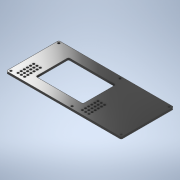
# Autodesk Inventor part: Sole_frame
Saved by Autodesk Inventor 2020.4 (Build 244396000, 396)
## iProperties
Part Number: Sole_frame
Material: GFRP
Document SubType Name: Modeling
Designer: Masato Kubotera
Density: 1.75 g/cm^3
Appearance: 低 光沢 - 黒
Description: GFRP T3
Mass: 61.6656 g
Surface Area: 261.936 cm^2
Volume: 35.2375 cm^3
Author: Masato Kubotera
Autodesk Inventor part; units mm, degrees
ref_plane "YZ Plane" through (0, 0, 0) normal (1, 0, 0) x (0, 1, 0)
ref_plane "XZ Plane" through (0, 0, 0) normal (0, 1, 0) x (-1, 0, 0)
ref_plane "XY Plane" through (0, 0, 0) normal (0, 0, 1) x (1, 0, 0)
sketch "スケッチ1" plane through (0, 0, 0) normal (0, 0, 1) x (1, 0, 0)
  line L0 (-96.735, 54.75) -> (78.265, 54.75)
  line L1 (78.265, 54.75) -> (78.265, -25.25)
  line L2 (78.265, -25.25) -> (-96.735, -25.25)
  line L3 (-96.735, -25.25) -> (-96.735, 54.75)
  line L4 (-96.735, 54.75) -> (78.265, -25.25) construction
  line L5 (78.265, 54.75) -> (-96.735, -25.25) construction
  line L6 (-96.735, 14.75) -> (78.265, 14.75) construction
  line L7 (-96.735, 0) -> (78.265, 0) construction
  line L8 (-80, 4.75) -> (-80, -4.75) construction
  circle A0 centre (-80, -4.75) radius 1.6
  line L9 (0, 54.75) -> (0, -25.25) construction
  line L10 (18, -4.75) -> (18, 4.75) construction
  circle A1 centre (18, -4.75) radius 1.6
  circle A2 centre (-80, 4.75) radius 1.6
  circle A3 centre (18, 4.75) radius 1.6
  line L11 (74.765, -21.75) -> (-93.235, -21.75) construction
  line L12 (-93.235, -21.75) -> (-93.235, 51.25) construction
  line L13 (-93.235, 51.25) -> (74.765, 51.25) construction
  line L14 (74.765, 51.25) -> (74.765, -21.75) construction
  line L15 (74.765, -21.75) -> (-93.235, 51.25) construction
  line L16 (-93.235, -21.75) -> (74.765, 51.25) construction
  circle A4 centre (-93.235, 51.25) radius 1.6
  circle A5 centre (0, 51.25) radius 1.6
  circle A6 centre (74.765, 51.25) radius 1.6
  circle A7 centre (-93.235, -21.75) radius 1.6
  circle A8 centre (0, -21.75) radius 1.6
  circle A9 centre (74.765, -21.75) radius 1.6
  line L17 (15, 12.5) -> (21, 12.5) construction
  line L18 (21, 12.5) -> (21, -12.5) construction
  line L19 (21, -12.5) -> (15, -12.5) construction
  line L20 (15, -12.5) -> (15, 12.5) construction
  line L21 (15, 12.5) -> (21, -12.5) construction
  line L22 (21, 12.5) -> (15, -12.5) construction
  line L23 (-83, 12.5) -> (-77, 12.5) construction
  line L24 (-77, 12.5) -> (-77, -12.5) construction
  line L25 (-77, -12.5) -> (-83, -12.5) construction
  line L26 (-83, -12.5) -> (-83, 12.5) construction
  line L27 (-83, 12.5) -> (-77, -12.5) construction
  line L28 (-77, 12.5) -> (-83, -12.5) construction
  line L29 (-67, 39.75) -> (5, 39.75)
  line L30 (5, 39.75) -> (5, -10.25)
  line L31 (5, -10.25) -> (-67, -10.25)
  line L32 (-67, -10.25) -> (-67, 39.75)
  line L33 (-67, 39.75) -> (5, -10.25) construction
  line L34 (5, 39.75) -> (-67, -10.25) construction
  circle A10 centre (-80, 0) radius 1.6
  circle A11 centre (18, 0) radius 1.6
  circle A12 centre (-80, -9.5) radius 1.6
  circle A13 centre (18, -9.5) radius 1.6
  circle A14 centre (-80, -4.75) radius 1.6
  circle A15 centre (18, -4.75) radius 1.6
  circle A16 centre (-80, -14.25) radius 1.6
  circle A17 centre (18, -14.25) radius 1.6
  circle A18 centre (-80, -9.5) radius 1.6
  circle A19 centre (18, -9.5) radius 1.6
  circle A20 centre (-80, -19) radius 1.6
  circle A21 centre (18, -19) radius 1.6
  circle A22 centre (-80, -14.25) radius 1.6
  circle A23 centre (18, -14.25) radius 1.6
  circle A24 centre (-85, 4.75) radius 1.6
  circle A25 centre (-85, 0) radius 1.6
  circle A26 centre (-85, -4.75) radius 1.6
  circle A27 centre (-85, -9.5) radius 1.6
  circle A28 centre (-85, -14.25) radius 1.6
  circle A29 centre (-85, -19) radius 1.6
  circle A30 centre (13, 4.75) radius 1.6
  circle A31 centre (13, 0) radius 1.6
  circle A32 centre (13, -4.75) radius 1.6
  circle A33 centre (13, -9.5) radius 1.6
  circle A34 centre (13, -14.25) radius 1.6
  circle A35 centre (13, -19) radius 1.6
  circle A36 centre (-75, 4.75) radius 1.6
  circle A37 centre (-75, 0) radius 1.6
  circle A38 centre (-75, -4.75) radius 1.6
  circle A39 centre (-75, -9.5) radius 1.6
  circle A40 centre (-75, -14.25) radius 1.6
  circle A41 centre (-75, -19) radius 1.6
  circle A42 centre (23, 4.75) radius 1.6
  circle A43 centre (23, 0) radius 1.6
  circle A44 centre (23, -4.75) radius 1.6
  circle A45 centre (23, -9.5) radius 1.6
  circle A46 centre (23, -14.25) radius 1.6
  circle A47 centre (23, -19) radius 1.6
  circle A48 centre (-80, 4.75) radius 1.6
  circle A49 centre (-80, 0) radius 1.6
  circle A50 centre (-80, -4.75) radius 1.6
  circle A51 centre (-80, -9.5) radius 1.6
  circle A52 centre (-80, -14.25) radius 1.6
  circle A53 centre (-80, -19) radius 1.6
  circle A54 centre (18, 4.75) radius 1.6
  circle A55 centre (18, 0) radius 1.6
  circle A56 centre (18, -4.75) radius 1.6
  circle A57 centre (18, -9.5) radius 1.6
  circle A58 centre (18, -14.25) radius 1.6
  circle A59 centre (18, -19) radius 1.6
  point P0 (0, 0)
  point P1 (-9.235, 14.75)
  point P2 (-80, 0)
  point P3 (18, 0)
  point P4 (-31, 14.75)
  dimension "d0" = 175
  dimension "d1" = 80
  dimension "d2" = 25.25
  dimension "d3" = 3.2
  dimension "d4" = 9.5
  dimension "d5" = 9.5
  dimension "d6" = 3.2
  dimension "d9" = 3.5
  dimension "d10" = 3.5
  dimension "d11" = 3.2
  dimension "d13" = 3.2
  dimension "d15" = 3.2
  dimension "d16" = 78.265
  dimension "d17" = 6
  dimension "d18" = 25
  dimension "d19" = 21
  dimension "d20" = 6
  dimension "d21" = 25
  dimension "d22" = 104
  dimension "d23" = 15
  dimension "d24" = 15
  dimension "d25" = 10
  dimension "d26" = 10
  dimension "d33" = 4.75
  dimension "d36" = 4.75
  dimension "d41" = 5
  dimension "d44" = 5
  constraints: 70 end point, 60 centre point, 14 midpoint, 10 parallel, 10 point on line, 7 horizontal, 7 perpendicular, 5 symmetric about line, 4 coincident, 4 vertical, 105 other
  measures "d0" distance of L1.end L2.end
  measures "d1" distance of L0.end L1.end
  measures "d2" distance of L2.end L7.start
  measures "d3" diameter of A0
  measures "d4" distance of L8.start L8.end
  measures "d5" distance of L10.start L10.end
  measures "d6" diameter of A1
  measures "d9" horizontal distance of L0.start L12.end
  measures "d10" horizontal distance of L0.start L12.end
  measures "d11" diameter of A4
  measures "d13" diameter of A5
  measures "d15" diameter of A6
  measures "d16" distance of L0.end L9.start
  measures "d17" distance of L18.end L19.end
  measures "d18" distance of L17.end L18.end
  measures "d19" horizontal distance of L17.end point (0, 0)
  measures "d20" distance of L24.end L25.end
  measures "d21" distance of L23.end L24.end
  measures "d22" distance of L18.end L25.end
  measures "d23" distance between parallel lines of L29 L0
  measures "d24" distance between parallel lines of L2 L31
  measures "d25" distance between parallel lines of L32 L24
  measures "d26" distance between parallel lines of L20 L30
  measures "d33" distance of A0.centre A10.centre
  measures "d36" distance of A0.centre A12.centre
  measures "d41" distance of A2.centre A24.centre
  measures "d44" distance of A2.centre A36.centre
extrude "押し出し1" add sketch "スケッチ1" along normal blind 3
fillet "フィレット1" radius 2 4 edges at (-96.735, 54.75, 1.5) (78.265, 54.75, 1.5) (78.265, -25.25, 1.5) (-96.735, -25.25, 1.5)
fillet "フィレット2" radius 2 4 edges at (-67, 39.75, 1.5) (-67, -10.25, 1.5) (5, -10.25, 1.5) (5, 39.75, 1.5)
equation "\"d3\" = d6"
equation "\"d4\" = d5"
equation "\"d10\" = d9"
equation "\"d11\" = d3"
equation "\"d13\" = d11"
equation "\"d15\" = d13"
equation "\"d20\" = d17"
equation "\"d21\" = d18"
equation "\"d33\" = 0.5 * d4"
equation "\"d36\" = 0.5 * d4"
equation "\"d41\" = d44"
